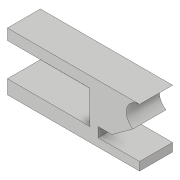
# Autodesk Inventor part: Halterung_MobileWhiteboard_V3
Saved by Autodesk Inventor 2017 (Build 210142000, 142)
## iProperties
Part Number: Halterung_MobileWhiteboard_V3
Material: Generisch
Document SubType Name: Modeling
Designer: Christoph Gürtner
Density: 1 g/cm^3
Appearance: Vorgabe
Author: Christoph Gürtner
Autodesk Inventor part; units mm, degrees
ref_plane "YZ Plane" through (0, 0, 0) normal (1, 0, 0) x (0, 1, 0)
ref_plane "XZ Plane" through (0, 0, 0) normal (0, 1, 0) x (-1, 0, 0)
ref_plane "XY Plane" through (0, 0, 0) normal (0, 0, 1) x (1, 0, 0)
sketch "Skizze1" plane through (0, 0, 0) normal (0, 1, 0) x (-1, 0, 0)
  arc A0 (4, -6.9282) -> (0, 8) centre (0, 0) ccw
  line L0 (0, -22) -> (0, -27)
  line L1 (0, -27) -> (30, -27)
  line L2 (80, 8) -> (0, 8)
  line L3 (0, -22) -> (25, -22)
  line L4 (25, -22) -> (0, -22)
  line L5 (25, -22) -> (25, -16.2)
  line L6 (25, -16) -> (25, -22)
  line L7 (25, -16.2) -> (16.7663, -16.2)
  line L8 (16.7663, -16.2) -> (4, -6.9282)
  line L9 (30, -27) -> (80, -27)
  line L10 (80, -27) -> (80, -18.6)
  line L11 (80, -18.6) -> (30, -18.6)
  line L12 (80, 8) -> (80, 1.45)
  line L13 (80, 1.45) -> (30, 1.45)
  line L14 (30, -18.6) -> (30, 1.45)
  dimension "d0" = 5
  dimension "d9" = 50
  dimension "d10" = 8.4
  dimension "d12" = 20.05
  constraints: 30 end point, 5 perpendicular, 4 horizontal, 4 vertical, 2 point on circle, 1 centre point, 1 coincident, 1 point on line, 2 other
  measures "d0" distance of L0.start L0.end
  measures "d9" distance of L1.end L9.end
  measures "d10" distance of L9.end L10.end
  measures "d12" distance between parallel lines of L13 L11
extrude "Extrusion1" add sketch "Skizze1" along normal blind 20
